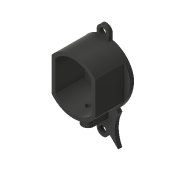
# Autodesk Inventor part: Motor Holder
Saved by Autodesk Inventor 2017 (Build 210142000, 142)
## iProperties
Created: 2016-10-10
Part Number: Motor Holder
Material: Generic
Document SubType Name: Modeling
Designer: ge937963
Density: 1 g/cm^3
Appearance: Smooth - Black
Author: ge937963
Autodesk Inventor part; units mm, degrees
ref_plane "YZ Plane" through (0, 0, 0) normal (1, 0, 0) x (0, 1, 0)
ref_plane "XZ Plane" through (0, 0, 0) normal (0, 1, 0) x (-1, 0, 0)
sketch "Sketch1" plane through (0, 0, 0) normal (0, 0, 1) x (1, 0, 0)
  line L0 (5.7396, -16.8109) -> (-2.4232, -6.7282) projected
  line L1 (-2.4232, -6.7282) -> (-8.3008, 0.7051) projected
  arc A0 (10.2494, 10.2845) -> (-8.3008, 0.7051) centre (0.0414, 7.3014) ccw projected
  arc A1 (2.7914, -3.3149) -> (10.2494, 10.2845) centre (0.2126, 6.944) ccw projected
  line L2 (2.7914, -3.3149) -> (5.9881, -7.541) projected
  arc A2 (6.711, -5.8652) -> (5.9881, -7.541) centre (19.909, -12.5525) ccw projected
  line L3 (6.711, -5.8652) -> (5.8177, -4.6842) projected
  arc A3 (5.8177, -4.6842) -> (11.7757, 8.697) centre (-6.2296, 8.697) ccw projected
  arc A4 (11.7757, 8.697) -> (2.54, 18.8513) centre (0.0414, 7.3014) ccw projected
  line L4 (-9.2281, -0.0281) -> (-2.54, -8.4863) projected
  line L5 (2.9614, -15.4438) -> (6.6502, -19.1185) projected
  arc A5 (5.7396, -16.8109) -> (6.6502, -19.1185) centre (19.909, -12.5525) ccw projected
  arc A6 (6.711, -5.8652) -> (6.6502, -19.1185) centre (19.909, -12.5525) ccw
  circle A7 centre (0.0414, 7.3014) radius 4.3509
  circle A8 centre (0, 21.4919) radius 1.27 projected
  line L6 (2.54, 18.8513) -> (2.54, 21.4919) projected
  arc A9 (2.54, 21.4919) -> (-2.54, 21.4919) centre (0, 21.4919) ccw projected
  line L7 (-2.54, 21.4919) -> (-2.54, 18.8331) projected
  arc A10 (-2.54, 18.8331) -> (-9.2281, -0.0281) centre (0.0414, 7.3014) ccw projected
  circle A11 centre (0, -15.0639) radius 1.27 projected
  line L8 (-2.54, -8.4863) -> (-2.54, -15.0639) projected
  arc A12 (-2.54, -15.0639) -> (2.54, -15.0639) centre (0, -15.0639) ccw projected
  line L9 (2.54, -15.0639) -> (2.54, -14.9108) projected
  line L10 (2.54, -14.9108) -> (2.9614, -15.4438) projected
  point P0 (0, 0)
  constraints: 3 point on circle, 2 centre point, 2 concentric
extrude "Extrusion1" add sketch "Sketch1" along normal blind 1.7 contours A5 L5 L10 L9 A12 L8 L4 A10 L7 A9 L6 A4 A3 L3 A2 L2 A1 A0 L1 L0 | L0 L1 A0 A1 L2 A6 | A8 | A11
sketch "Sketch2" plane through (0, 0, 1.7) normal (0, 0, 1) x (1, 0, 0)
  circle A0 centre (0, 21.4919) radius 1.524
  circle A1 centre (0, -15.0639) radius 1.524
  line L0 (2.54, 17.6957) -> (-2.54, 17.6957)
  line L1 (-2.54, 17.6957) -> (-2.54, 21.4919)
  line L2 (2.54, 17.6957) -> (2.54, 21.4919)
  arc A2 (2.54, 21.4919) -> (-2.54, 21.4919) centre (0, 21.4919) ccw
  arc A3 (-2.54, -15.0639) -> (2.54, -15.0639) centre (0, -15.0639) ccw
  line L3 (-2.54, -15.0639) -> (-2.54, -7.1979)
  line L4 (-2.54, -7.1979) -> (2.54, -12.2319)
  line L5 (2.54, -12.2319) -> (2.54, -15.0639)
  point P0 (0, 0)
  dimension "d2" = 3.048
  dimension "d3" = 3.048
  dimension "d4" = 2.54
  dimension "d5" = 2.54
  constraints: 12 end point, 4 centre point, 4 point on circle, 2 collinear, 2 concentric, 2 tangent, 2 vertical, 1 horizontal, 1 perpendicular, 1 vertical alignment
  measures "d2" diameter of A0
  measures "d3" diameter of A1
  measures "d4" radius of A2
  measures "d5" radius of A3
ref_plane "Work Plane1" through (-11.7757, -19.1185, 0) normal (0, 0, 1) x (1, 0, 0)
sketch "Sketch3" plane through (0, 0, 1.7) normal (0, 0, 1) x (1, 0, 0)
  line L0 (-7.5086, 0.6681) -> (-7.5086, 13.9346) projected
  arc A0 (7.5914, 13.9346) -> (-7.5086, 13.9346) centre (0.0414, 7.3014) ccw projected
  arc A1 (-7.5086, 0.6681) -> (7.5914, 0.6681) centre (0.0414, 7.3014) ccw projected
  line L1 (7.5914, 13.9346) -> (7.5914, 0.6681) projected
  arc A2 (-7.7626, 0.5731) -> (7.8454, 0.5731) centre (0.0414, 7.3014) ccw
  line L2 (-7.7626, 0.5731) -> (-7.7626, 14.0297)
  arc A3 (7.8454, 14.0297) -> (-7.7626, 14.0297) centre (0.0414, 7.3014) ccw
  line L3 (7.8454, 14.0297) -> (7.8454, 0.5731)
  arc A4 (-9.2757, 0.0326) -> (9.3585, 0.0326) centre (0.0414, 7.3014) ccw
  line L4 (-9.2757, 0.0326) -> (-9.2757, 14.5702)
  arc A5 (9.3585, 14.5702) -> (-9.2757, 14.5702) centre (0.0414, 7.3014) ccw
  line L5 (9.3585, 14.5702) -> (9.3585, 0.0326)
  line L6 (-9.2281, -0.0281) -> (-2.54, -8.4863) projected
  line L7 (2.9614, -15.4438) -> (6.6502, -19.1185) projected
  arc A6 (6.711, -5.8652) -> (6.6502, -19.1185) centre (19.909, -12.5525) ccw projected
  line L8 (6.711, -5.8652) -> (5.8177, -4.6842) projected
  arc A7 (5.8177, -4.6842) -> (11.7757, 8.697) centre (-6.2296, 8.697) ccw projected
  arc A8 (11.7757, 8.697) -> (2.54, 18.8513) centre (0.0414, 7.3014) ccw projected
  circle A9 centre (0.0414, 7.3014) radius 4.3509 projected
  arc A10 (11.7757, 8.697) -> (2.54, 18.8513) centre (0.0414, 7.3014) ccw projected
  line L9 (2.54, 18.8513) -> (2.54, 21.4919) projected
  arc A11 (2.54, 21.4919) -> (-2.54, 21.4919) centre (0, 21.4919) ccw projected
  line L10 (-2.54, 21.4919) -> (-2.54, 18.8331) projected
  arc A12 (-2.54, 18.8331) -> (-9.2281, -0.0281) centre (0.0414, 7.3014) ccw projected
  line L11 (-2.54, -8.4863) -> (-2.54, -15.0639) projected
  arc A13 (-2.54, -15.0639) -> (2.54, -15.0639) centre (0, -15.0639) ccw projected
  line L12 (2.54, -15.0639) -> (2.54, -14.9108) projected
  line L13 (2.54, -14.9108) -> (2.9614, -15.4438) projected
  point P0 (0, 0)
  dimension "d8" = 0.254
  constraints: 9 point on circle, 8 end point, 4 centre point, 6 other
  measures "d8" distance between parallel lines of L1 L3
extrude "Extrusion3" add sketch "Sketch3" along normal blind 12.7 contours L4 A5 L5 A4
extrude "Extrusion4" cut sketch "Sketch2" against normal blind 12.7 contours A0 | A1
sketch "Sketch4" plane through (0, 0, 0) normal (0, 1, 0) x (-1, 0, 0)
  line L0 (9.2757, 14.4) -> (-9.3585, 14.4) projected
  line L1 (9.2757, 1.7) -> (9.2757, 14.4) projected
  line L2 (-9.3585, 1.7) -> (-9.3585, 14.4) projected
  line L3 (2.54, 1.7) -> (-2.54, 1.7) projected
  line L4 (2.54, 1.7) -> (-2.54, 1.7) projected
  line L5 (2.54, 1.7) -> (2.54, 8.05)
  line L6 (-2.54, 1.7) -> (-2.54, 8.05)
  arc A0 (2.54, 8.05) -> (-2.54, 8.05) centre (0, 8.05) ccw
  point P0 (0, 0)
  point P1 (-9.3585, 8.05)
  constraints: 5 end point, 2 horizontal alignment, 2 point on circle, 2 vertical, 1 centre point, 1 midpoint, 1 tangent
extrude "Extrusion5" add sketch "Sketch4" against normal blind 9.525
sketch "Sketch5" plane through (0, 0, 14.4) normal (0, 0, 1) x (1, 0, 0)
  line L0 (-7.7626, 0.5731) -> (-7.7626, 14.0297) projected
  arc A0 (7.8454, 14.0297) -> (-7.7626, 14.0297) centre (0.0414, 7.3014) ccw projected
  line L1 (7.8454, 14.0297) -> (7.8454, 0.5731) projected
  arc A1 (-7.7626, 0.5731) -> (7.8454, 0.5731) centre (0.0414, 7.3014) ccw projected
  line L2 (9.3585, 0.0326) -> (9.3585, 14.5702) projected
  arc A2 (9.3585, 14.5702) -> (-9.2757, 14.5702) centre (0.0414, 7.3014) ccw projected
  line L3 (-9.2757, 14.5702) -> (-9.2757, 0.0326) projected
  arc A3 (-9.2757, 0.0326) -> (9.3585, 0.0326) centre (0.0414, 7.3014) ccw projected
  point P0 (0, 0)
extrude "Extrusion6" cut sketch "Sketch5" against normal up to surface (12.7 mm away) contours L0 A0 L1 A1
sketch "Sketch6" plane through (0, -9.525, 0) normal (0, -1, 0) x (1, 0, 0)
  circle A0 centre (0, 8.05) radius 1.016
  arc A1 (2.54, 8.05) -> (-2.54, 8.05) centre (0, 8.05) ccw projected
  point P0 (0, 0)
  dimension "d17" = 2.032
  constraints: 1 centre point, 1 concentric
  measures "d17" diameter of A0
extrude "Extrusion7" cut sketch "Sketch6" against normal blind 12.7
body "Solid1"
